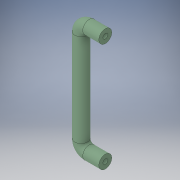
# Autodesk Inventor part: Rubber pipe turn
Saved by Autodesk Inventor 2019 (Build 230136000, 136)
## iProperties
Created: 2019-06-27
Part Number: Rubber pipe turn
Material: Generic
Document SubType Name: Sheet Metal
Designer: Satwik Pandey
Density: 1 g/cm^3
Sheet Metal Rule: Default_mm
Appearance: Rubber - Green
Author: Satwik Pandey
Autodesk Inventor part; units mm, degrees
ref_plane "YZ Plane" through (0, 0, 0) normal (1, 0, 0) x (0, 1, 0)
ref_plane "XZ Plane" through (0, 0, 0) normal (0, 1, 0) x (-1, 0, 0)
ref_plane "XY Plane" through (0, 0, 0) normal (0, 0, 1) x (1, 0, 0)
sketch "Sketch3" plane through (0, 0, 0) normal (1, 0, 0) x (0, 1, 0)
  circle A0 centre (0, 0) radius 8
  circle A1 centre (0, 0) radius 3
  dimension "d4" = 16
  dimension "d5" = 6
  constraints: 2 centre point, 2 coincident
  measures "d4" diameter of A0
  measures "d5" diameter of A1
sketch "Sketch4" plane through (0, 0, 0) normal (0, 0, 1) x (1, 0, 0)
  line L0 (0, 0) -> (-20, 0)
  line L1 (-30, -10) -> (-30, -96)
  arc A0 (-20, 0) -> (-30, -10) centre (-20, -10) ccw
  line L2 (0, -134.8) -> (-20, -134.8)
  line L3 (-20, -134.8) -> (-20, -134.8)
  line L4 (-30, -124.8) -> (-30, -96)
  arc A1 (-30, -124.8) -> (-20, -134.8) centre (-20, -124.8) ccw
  point P0 (-30, -106)
  point P1 (-30, -134.8)
  constraints: 10 end point, 4 point on circle, 4 point on line, 4 tangent, 2 centre point, 2 horizontal, 1 perpendicular, 1 vertical
sweep "Sweep2" add profiles "Sketch3" path "Sketch4"
equation "\"BendRadius\" = Thickness"
equation "\"BendReliefWidth\" = Thickness"
equation "\"BendReliefDepth\" = 0.5 * Thickness"
equation "\"CornerReliefSize\" = 4 * Thickness"
equation "\"MinimumRemnant\" = 2 * Thickness"
equation "\"TransitionRadius\" = BendRadius"
equation "\"JacobiRadiusSize\" = BendRadius"
equation "\"GapSize\" = Thickness"
equation "\"Thickness\" = 0.5"
body "Solid2"
